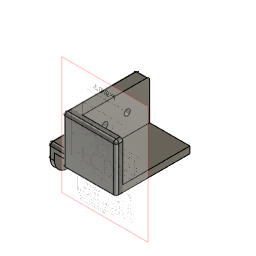
side-mount-rear v3 (Autodesk Fusion 360 design; units mm, degrees)
Autodesk Fusion 360 part; units mm, degrees
note: some values were not read from the file. Chosen so that the rebuilt part matches the saved one: which pieces of a blend or face edit are solid.
sketch "Sketch3" plane through (0, 0, 0) normal (0, 1, 0) x (1, 0, 0)
  line L0 (-15, -15) -> (15, -15)
  line L1 (15, -15) -> (15, 15)
  line L2 (15, 15) -> (-15, 15)
  line L3 (-15, 15) -> (-15, -15)
  dimension "d5" = 30
  dimension "d6" = 30
  dimension "d7" = 15
  dimension "d8" = 15
  constraint horizontal L0
  constraint vertical L1
  constraint horizontal L2
  constraint vertical L3
  measures "d5" distance of L0.start L0.end
  measures "d6" distance of L0.start L2.end
  measures "d7" distance of origin L0
  measures "d8" distance of origin L3
sketch "Sketch1" plane through (0, 0, 0) normal (0, 1, 0) x (1, 0, 0) in component "Component'"
  line L0 (-25, -15) -> (-15, -15)
  line L1 (-15, -15) -> (-15, 15)
  line L2 (-15, 15) -> (15, 15)
  line L3 (15, 15) -> (15, 20)
  line L4 (15, 20) -> (-36, 20)
  line L5 (-36, 20) -> (-36, 35)
  line L6 (-36, 35) -> (-41, 35)
  line L7 (-41, 35) -> (-41, 15)
  line L8 (-41, 15) -> (-25, 15)
  line L9 (-25, 15) -> (-25, -15)
  dimension "d15" = 10
  dimension "d16" = 5
  constraint horizontal L0
  constraint perpendicular L0 L1
  constraint perpendicular L1 L2
  constraint perpendicular L2 L3
  constraint perpendicular L3 L4
  constraint perpendicular L4 L5
  constraint perpendicular L5 L6
  constraint perpendicular L6 L7
  constraint perpendicular L7 L8
  constraint perpendicular L0 L9
  constraint coincident L7.end L8.start
  measures "d15" distance of L1 L9
  measures "d16" distance of L5 L7
extrude "Extrude1" add sketch "Sketch1" along normal blind 50 makes body 1 in component "Component'"
sketch "Sketch3 (2)" plane through (-25, 0, 0) normal (-1, 0, 0) x (0, -1, 0) in component "Component'"
  line L0 (0, -15) -> (0, 15)
  line L1 (0, 15) -> (-50, 15)
  line L2 (-50, 15) -> (-50, -15)
  line L3 (-50, -15) -> (0, -15)
  point P0 (-33.3333, 0)
  point P1 (-16.6667, 0)
  dimension "d30" = 16.6667
  dimension "d31" = 16.6667
  measures "d30" distance of L2 P0
  measures "d31" distance of P0 P1
hole "Hole2" at (-25, 33.3333, 0) at (-25, 16.6667, 0) direction (1, 0, 0) diameter 4.5 depth 12 tip angle 118 counterbore diameter 8 counterbore depth 4.6 bodies 1 in component "Component'"
sketch "Sketch4" plane through (0, 0, 0) normal (0, -1, 0) x (1, 0, 0) in component "Component'"
  line L0 (-25, 15) -> (-25, -15)
  line L1 (-25, -15) -> (-41, -15)
  line L2 (-41, -15) -> (-41, -35)
  line L3 (-41, -35) -> (-36, -35)
  line L4 (-36, -35) -> (-36, -20)
  line L5 (-36, -20) -> (15, -20)
  line L6 (15, -20) -> (15, -15)
  line L7 (15, -15) -> (-15, -15)
  line L8 (-15, -15) -> (-15, 15)
  line L9 (-15, 15) -> (-25, 15)
  line L10 (-25, 15) -> (15, 15)
  line L11 (15, 15) -> (15, -20)
  line L12 (15, -20) -> (-25, -20)
  line L13 (-25, -20) -> (-25, 15)
  constraint horizontal L10
  constraint vertical L11
  constraint horizontal L12
  constraint vertical L13
  constraint coincident L5.end L6.start
  constraint coincident L0.start L9.end
extrude "Extrude2" add sketch "Sketch4" along normal blind 5 contours L0 L5 L6 L7 L8 L9 L10 L11 L12 L13 | L7 L8 L10 L11 bodies 1 in component "Component'"
imported_body "Base Feature1" makes body 2 in component "le-6-gb3030"
sketch "Sketch7" plane through (0, 0, 0) normal (0, 1, 0) x (-1, 0, 0)
  line L0 (15, -15) -> (15, 15)
  line L1 (15, 15) -> (-15, 15)
  line L2 (-15, 15) -> (-15, -15)
  line L3 (-15, -15) -> (15, -15)
  line L4 (-4, -15) -> (-4, -13)
  line L5 (-4, -13) -> (-8, -13)
  line L6 (-8, -13) -> (-8, -10)
  line L7 (-8, -10) -> (-4.5, -6)
  line L8 (-4.5, -6) -> (4.5, -6)
  line L9 (4.5, -6) -> (8, -10)
  line L10 (8, -10) -> (8, -13)
  line L11 (8, -13) -> (4, -13)
  line L12 (4, -13) -> (4, -15)
  line L13 (0, -3.1113) -> (0, -18.5) construction
  dimension "d81" = 8
  dimension "d82" = 4
  dimension "d84" = 8
  dimension "d85" = 3
  dimension "d86" = 9
  dimension "d87" = 2
  dimension "d89" = 4.5
  dimension "d90" = 9
  dimension "d91" = 2
  dimension "d92" = 16
  dimension "d93" = 3
  constraint coincident L3 L4.start
  constraint perpendicular L3 L4
  constraint perpendicular L4 L5
  constraint perpendicular L5 L6
  constraint perpendicular L6 L8
  constraint parallel L6 L10
  constraint perpendicular L10 L11
  constraint coincident L3 L12.end
  constraint perpendicular L3 L12
  constraint vertical L13
  constraint coincident origin L13
  measures "d81" distance of L4.start L12.end
  measures "d82" distance of L4 L13
  measures "d84" distance of L5.end L13
  measures "d85" distance of L5.end L6.end
  measures "d86" distance of L7.end L8.end
  measures "d87" distance of L4.start L4.end
  measures "d89" distance of L7.end L13
  measures "d90" distance of L8 L12.end
  measures "d91" distance of L11.end L12.end
  measures "d92" distance of L5.end L10.end
  measures "d93" distance of L9.end L10.end
fillet "Fillet4" radius 2 7 edges at (15, -5, -2.5) (-5, -5, 15) (-25, -5, -2.5) (-25, 22.5, 15) (-25, 50, 0) (-20, 50, 15) (15, -2.5, 15) on bodies 1 in component "Component'"
fillet "Fillet5" radius 10 2 edges at (-38.5, 50, -35) (-38.5, 0, -35) on bodies 1 in component "Component'"
fillet "Fillet6" radius 2 8 edges at (-32, 50, -15) (-41, 0, -20) (-41, 2.9289, -32.0711) (-41, 25, -35) (-41, 47.0711, -32.0711) (-41, 50, -20) (-33, 0, -15) (-41, 25, -15) on bodies 1 in component "Component'"
fillet "Fillet6" radius 2 1 edges at (-25, 0, -17.5) on bodies 1 in component "Component'"
component "Component" placed x (1, 0, 0) y (0, 1, 0) z (0, 0, 1) at (0, 0, 0)
component "Component'" placed x (1, 0, 0) y (0, 1, 0) z (0, 0, 1) at (0, 0, 0)
component "le-6-gb3030" placed x (1, 0, 0) y (0, 0, 1) z (0, -1, 0) at (3297.6791, 50.0607, -3567.1588)
hidden bodies 2
equation "d30 = ( 50 / 3 ) * 1 mm"
equation "d31 = d30"
equation "d82 = d81 / 2"
